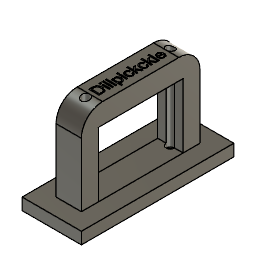
HANDLE (Autodesk Fusion 360 design; units mm, degrees)
Autodesk Fusion 360 part; units mm, degrees
sketch "Sketch1" plane through (0, 0, 0) normal (0, 0, 1) x (1, 0, 0)
  line L0 (0, 0) -> (35, 0)
  line L1 (35, 0) -> (35, -90)
  line L2 (35, -90) -> (0, -90)
  line L3 (0, -90) -> (0, 0)
  dimension "d1" = 35
  dimension "d2" = 90
  constraint horizontal L0
  constraint vertical L1
  constraint horizontal L2
  constraint vertical L3
  constraint coincident L0.start L3.end
  measures "d1" distance of L0.start L0.end
  measures "d2" distance of L0.start L2.end
extrude "Extrude1" add sketch "Sketch1" along normal blind 7
sketch "Sketch2" plane through (0, 0, 7) normal (0, 0, 1) x (-1, 0, 0)
  line L0 (0, 90) -> (-35, 90)
  line L1 (-35, 90) -> (-35, 0)
  line L2 (-35, 0) -> (0, 0)
  line L3 (0, 0) -> (0, 90)
  circle A0 centre (-17.5, 20) radius 1.5
  circle A1 centre (-17.5, 70) radius 1.5
  circle A2 centre (-17.5, 20) radius 2.5
  circle A3 centre (-17.5, 70) radius 2.5
  dimension "d6" = 3
  dimension "d7" = 3
  dimension "d8" = 17.5
  dimension "d9" = 17.5
  dimension "d10" = 20
  dimension "d11" = 20
  dimension "d12" = 5
  dimension "d13" = 5
  constraint concentric A0 A2
  constraint concentric A1 A3
  measures "d6" diameter of A0
  measures "d7" diameter of A1
  measures "d8" distance of L3 A0.centre
  measures "d9" distance of L3 A1.centre
  measures "d10" distance of L0 A1.centre
  measures "d11" distance of L2 A0.centre
  measures "d12" diameter of A2
  measures "d13" diameter of A3
extrude "Extrude2" cut sketch "Sketch2" against normal blind 2.5 contours A2 | A3
extrude "Extrude3" cut 2 faces at (17.9131, -69.4236, 7) (17.8938, -19.2956, 7) along direction (0, 0, -1) blind 7
sketch "Sketch3" plane through (0, 0, 7) normal (0, 0, 1) x (-1, 0, 0)
  circle A0 centre (-17.5, 20) radius 2.5
  circle A1 centre (-17.5, 70) radius 2.5
  line L0 (0, 90) -> (-35, 90)
  line L1 (-35, 90) -> (-35, 0)
  line L2 (-35, 0) -> (0, 0)
  line L3 (0, 0) -> (0, 90)
sketch "Sketch4" plane through (0, 0, 0) normal (1, 0, 0) x (0, 1, 0)
sketch "Sketch5" plane through (0, 0, 7) normal (0, 0, 1) x (-1, 0, 0)
  line L0 (-25, 10) -> (-10, 10)
  line L1 (-10, 10) -> (-10, 80)
  line L2 (-10, 80) -> (-25, 80)
  line L3 (-25, 80) -> (-25, 10)
  constraint horizontal L0
  constraint vertical L1
  constraint horizontal L2
  constraint vertical L3
extrude "Extrude4" add sketch "Sketch5" along normal blind 50
sketch "Sketch6" plane through (10, 0, 0) normal (-1, 0, 0) x (0, -1, 0)
  line L0 (10, 7) -> (80, 7)
  line L1 (80, 7) -> (80, 57)
  line L2 (80, 57) -> (10, 57)
  line L3 (10, 57) -> (10, 7)
  line L4 (15, 7) -> (74.857, 7)
  line L5 (20, 45) -> (70, 45)
  line L6 (70, 45) -> (70, 7)
  line L7 (20, 7) -> (20, 45)
  constraint coincident L0 L4.start
  constraint coincident L0 L4.end
  constraint parallel L2 L5
  constraint coincident L4 L6.end
  constraint perpendicular L4 L6
  constraint coincident L4 L7.start
extrude "Extrude5" cut sketch "Sketch6" against normal blind 15 contours L0 L4 L5 L6 L7
fillet "Fillet1" radius 12.5 2 edges at (17.5, -10, 57) (17.5, -80, 57)
extrude "Extrude6" cut sketch "Sketch3" along normal blind 55 contours A0 | A1
sketch "Sketch7" plane through (0, 0, 57) normal (0, 0, 1) x (-1, 0, 0)
  line L0 (-17.5, 67.5) -> (-25, 67.5)
  line L1 (-25, 67.5) -> (-25, 22.5)
  line L2 (-25, 22.5) -> (-17.5, 22.5)
  line L3 (-17.5, 22.5) -> (-10, 22.5)
  line L4 (-10, 22.5) -> (-10, 67.5)
  line L5 (-10, 67.5) -> (-17.5, 67.5)
  line L6 (-40.1656, 52.3344) -> (-40.1656, 37.6656) construction
  line L7 (-40.1656, 37.6656) -> (4.8344, 37.6656) construction
  line L8 (4.8344, 37.6656) -> (4.8344, 52.3344) construction
  line L9 (4.8344, 52.3344) -> (-40.1656, 52.3344) construction
  dimension "d26" = 6
  text T0 "Dillpickckle" font "Arial" height 6 align centre middle in box 14.6688 x 45 at (-40.1656, 52.3344) x (0, -1) y (1, 0) spacing 1
extrude "Extrude7" cut sketch "Sketch7" against normal blind 2.5 text T0
equation "d27 = 'Dillpickckle'"
